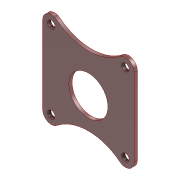
# Autodesk Inventor part: seal
Saved by Autodesk Inventor 2020 (Build 240168000, 168)
## iProperties
Created: 2020-05-08
Part Number: seal
Material: Generic
Document SubType Name: Modeling
Designer: rayan
Density: 1 g/cm^3
Appearance: LED - Red Off
Author: rayan
Autodesk Inventor part; units mm, degrees
ref_plane "YZ Plane" through (0, 0, 0) normal (1, 0, 0) x (0, 1, 0)
ref_plane "XZ Plane" through (0, 0, 0) normal (0, 1, 0) x (-1, 0, 0)
ref_plane "XY Plane" through (0, 0, 0) normal (0, 0, 1) x (1, 0, 0)
sketch "Sketch3" plane through (0, 0, 0) normal (0, 0, 1) x (1, 0, 0)
  line L0 (-20.1, 21) -> (20.1, 21)
  line L1 (20.1, 21) -> (20.1, -21)
  line L2 (20.1, -21) -> (-20.1, -21)
  line L3 (-20.1, -21) -> (-20.1, 21)
  line L4 (-20.1, 21) -> (20.1, -21) construction
  line L5 (20.1, 21) -> (-20.1, -21) construction
  point P0 (0, 0)
  dimension "d24" = 40.2
  dimension "d25" = 42
  constraints: 12 end point, 2 midpoint, 2 parallel, 1 horizontal, 1 perpendicular
  measures "d24" distance of L1.end L2.end
  measures "d25" distance of L0.end L1.end
extrude "Extrusion3" add sketch "Sketch3" along normal blind 1.5
sketch "Sketch4" plane through (0, 0, 1.5) normal (0, 0, 1) x (1, 0, 0)
  line L0 (20.1, 21) -> (-20.1, 21) projected
  line L1 (-20.1, 21) -> (-17.1, 21) construction
  line L2 (-17.1, 21) -> (-17.1, 18) construction
  line L3 (-17.1, 18) -> (-20.1, 18) construction
  line L4 (-20.1, 18) -> (-20.1, 21) construction
  circle A0 centre (-17.1, 18) radius 1.7
  point P0 (0, 0)
  dimension "d28" = 3
  dimension "d29" = 3
  dimension "d30" = 3.4
  constraints: 8 end point, 2 parallel, 1 centre point, 1 coincident, 1 horizontal, 1 perpendicular
  measures "d28" distance of L2.end L3.end
  measures "d29" distance of L1.end L2.end
  measures "d30" diameter of A0
extrude "Extrusion4" cut sketch "Sketch4" against normal through all
fillet "Fillet2" radius 3 1 edges at (-20.1, 21, 0.75)
mirror "Mirror2" about plane through (0, 0, 0) normal (0, 1, 0) of "Fillet2", "Extrusion4"
mirror "Mirror3" about plane through (0, 0, 0) normal (1, 0, 0) of "Fillet2", "Extrusion4", "Mirror2"
sketch "Sketch5" plane through (0, 0, 1.5) normal (0, 0, 1) x (1, 0, 0)
  circle A0 centre (-17.1, 18) radius 1.7 construction
  circle A1 centre (17.1, 18) radius 1.7 construction
  line L0 (-17.1, 18) -> (17.1, 18) construction
  line L1 (17.1, 18) -> (17.1, 15) construction
  line L2 (17.1, 15) -> (-17.1, 15) construction
  line L3 (-17.1, 15) -> (-17.1, 18) construction
  arc A2 (-17.1, 21) -> (-20.1, 18) centre (-17.1, 18) ccw projected
  line L4 (-17.1, 18) -> (-17.1, 21) construction
  line L5 (17.1, 21) -> (-17.1, 21) construction
  line L6 (17.1, 18) -> (17.1, 21) construction
  arc A3 (20.1, 18) -> (17.1, 21) centre (17.1, 18) ccw construction
  line L7 (17.1, 21) -> (-17.1, 21) construction
  line L8 (-17.1, 18) -> (-17.1, 21) construction
  line L9 (-17.1, 21) -> (-16, 21) construction
  line L10 (-16, 21) -> (-16, 18) construction
  line L11 (-16, 18) -> (-17.1, 18) construction
  line L12 (17.1, 18) -> (17.1, 21) construction
  line L13 (17.1, 21) -> (16, 21) construction
  line L14 (16, 21) -> (16, 18) construction
  line L15 (16, 18) -> (17.1, 18) construction
  arc A4 (-16, 21) -> (16, 21) centre (0, 39.3333) ccw
  line L16 (-16, 21) -> (16, 21)
  point P0 (0, 0)
  point P1 (0, 15)
  dimension "d34" = 3
  dimension "d42" = 1.1
  dimension "d43" = 1.1
  constraints: 30 end point, 6 parallel, 4 perpendicular, 3 point on circle, 2 collinear, 2 vertical, 1 centre point, 1 horizontal, 1 midpoint
  measures "d34" distance of L0.end L1.end
  measures "d42" distance of L4.end L9.end
  measures "d43" distance of L5.start L13.end
extrude "Extrusion5" cut sketch "Sketch5" against normal through all
mirror "Mirror4" about plane through (0, 0, 0) normal (0, 1, 0) of "Extrusion5"
fillet "Fillet3" radius 3 4 edges at (-16, 21, 0.75) (16, 21, 0.75) (16, -21, 0.75) (-16, -21, 0.75)
sketch "Sketch7" plane through (0, 0, 1.5) normal (0, 0, 1) x (1, 0, 0)
  line L0 (15.3, 7.9) -> (15.3, -11.6) construction
  line L1 (15.3, -11.6) -> (-15.4, -11.6) construction
  line L2 (-15.4, -11.6) -> (-15.4, 7.9) construction
  line L3 (-15.4, 7.9) -> (15.3, 7.9) construction
  line L4 (-17.65, -15) -> (30.6, -15) construction
  line L5 (30.6, -15) -> (30.6, 15) construction
  line L6 (30.6, 15) -> (-30.1, 15) construction
  line L7 (-30.1, 15) -> (-30.1, 10) construction
  line L8 (-17.65, 10) -> (-30.1, 10) construction
  line L9 (-17.65, 10) -> (-17.65, -15) construction
  line L10 (15.3, -11.6) -> (-15.4, 7.9) construction
  line L11 (-15.4, -11.6) -> (15.3, 7.9) construction
  line L12 (0, 0) -> (-0.05, 0) construction
  line L13 (-0.05, 0) -> (-0.05, -1.85) construction
  line L14 (-0.05, -1.85) -> (0, -1.85) construction
  line L15 (0, -1.85) -> (0, 0) construction
  circle A0 centre (0, -1.85) radius 9
  dimension "d41" = 18
  constraints: 12 end point, 2 parallel, 1 centre point, 1 coincident, 1 horizontal, 1 midpoint, 1 perpendicular
  measures "d41" diameter of A0
extrude "Extrusion6" cut sketch "Sketch7" against normal through all
sketch "Sketch8" plane through (0, 0, 1.5) normal (0, 0, 1) x (1, 0, 0)
  circle A0 centre (0, -1.85) radius 9 projected
  arc A1 (-17.088, -21) -> (-15.2125, -20.3415) centre (-17.088, -18) ccw projected
  arc A2 (15.2125, -20.3415) -> (-15.2125, -20.3415) centre (0, -39.3333) ccw projected
  arc A3 (15.2125, -20.3415) -> (17.088, -21) centre (17.088, -18) ccw projected
  line L0 (17.088, -21) -> (17.1, -21) projected
  arc A4 (17.1, -21) -> (20.1, -18) centre (17.1, -18) ccw projected
  line L1 (20.1, -18) -> (20.1, 18) projected
  arc A5 (20.1, 18) -> (17.1, 21) centre (17.1, 18) ccw projected
  line L2 (17.1, 21) -> (17.088, 21) projected
  arc A6 (17.088, 21) -> (15.2125, 20.3415) centre (17.088, 18) ccw projected
  arc A7 (-15.2125, 20.3415) -> (15.2125, 20.3415) centre (0, 39.3333) ccw projected
  arc A8 (-15.2125, 20.3415) -> (-17.088, 21) centre (-17.088, 18) ccw projected
  line L3 (-17.088, 21) -> (-17.1, 21) projected
  arc A9 (-17.1, 21) -> (-20.1, 18) centre (-17.1, 18) ccw projected
  line L4 (-20.1, 18) -> (-20.1, -18) projected
  arc A10 (-20.1, -18) -> (-17.1, -21) centre (-17.1, -18) ccw projected
  line L5 (-17.1, -21) -> (-17.088, -21) projected
  circle A11 centre (17.1, -18) radius 1.7 projected
  circle A12 centre (17.1, 18) radius 1.7 projected
  circle A13 centre (-17.1, -18) radius 1.7 projected
  circle A14 centre (-17.1, 18) radius 1.7 projected
  line L6 (21.1, 18) -> (21.1, -18)
  arc A15 (17.1, -22) -> (21.1, -18) centre (17.1, -18) ccw
  line L7 (17.1, -22) -> (17.088, -22)
  arc A16 (14.5873, -21.122) -> (17.088, -22) centre (17.088, -18) ccw
  arc A17 (14.5873, -21.122) -> (-14.5873, -21.122) centre (0, -39.3333) ccw
  arc A18 (-17.088, -22) -> (-14.5873, -21.122) centre (-17.088, -18) ccw
  line L8 (-17.088, -22) -> (-17.1, -22)
  arc A19 (-21.1, -18) -> (-17.1, -22) centre (-17.1, -18) ccw
  line L9 (-21.1, -18) -> (-21.1, 18)
  arc A20 (-17.1, 22) -> (-21.1, 18) centre (-17.1, 18) ccw
  line L10 (-17.1, 22) -> (-17.088, 22)
  arc A21 (-14.5873, 21.122) -> (-17.088, 22) centre (-17.088, 18) ccw
  arc A22 (-14.5873, 21.122) -> (14.5873, 21.122) centre (0, 39.3333) ccw
  arc A23 (17.088, 22) -> (14.5873, 21.122) centre (17.088, 18) ccw
  line L11 (17.088, 22) -> (17.1, 22)
  arc A24 (21.1, 18) -> (17.1, 22) centre (17.1, 18) ccw
  point P0 (0, 0)
  dimension "d44" = 1
  constraints: 20 point on circle, 12 end point, 10 centre point, 15 other
  measures "d44" distance between parallel lines of L1 L6
extrude "Extrusion7" add sketch "Sketch8" against normal up to surface (1.5 mm away) contours L6 A15 L7 A16 A17 A18 L8 A19 L9 A20 L10 A21 A22 A23 L11 A24
equation "\"d43\" = d42"
body "Solid2"
